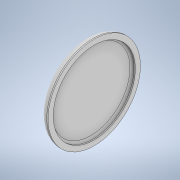
# Autodesk Inventor part: Регулировка-тихая
Saved by Autodesk Inventor 2021 (Build 250183000, 183)
## iProperties
Created: 2023-04-26
Part Number: Регулировка-тихая
Material: Типовые
Document SubType Name: Modeling
Designer: gdevc
Density: 1 g/cm^3
Appearance: По умолчанию
Mass: 33.1576 g
Surface Area: 146.506 cm^2
Volume: 33.1576 cm^3
Author: gdevc
Autodesk Inventor part; units mm, degrees
ref_plane "YZ Plane" through (0, 0, 0) normal (1, 0, 0) x (0, 1, 0)
ref_plane "XZ Plane" through (0, 0, 0) normal (0, 1, 0) x (-1, 0, 0)
ref_plane "XY Plane" through (0, 0, 0) normal (0, 0, 1) x (1, 0, 0)
sketch "Эскиз1" plane through (0, 0, 0) normal (0, 0, 1) x (1, 0, 0)
  line L0 (0, 0) -> (29.6206, 0)
  line L1 (0, 0) -> (0, 38)
  line L2 (2, 40) -> (3.25, 40)
  arc A0 (2, 40) -> (0, 38) centre (2, 38) ccw
  line L3 (3.25, 45) -> (2, 45)
  arc A1 (2, 45) -> (-5, 38) centre (2, 38) ccw
  line L4 (-5, 38) -> (-5, 0)
  line L5 (-5, 0) -> (0, 0)
  line L6 (3.25, 45) -> (3.25, 40)
  dimension "d0" = 80
  dimension "d1" = 2
  dimension "d2" = 90
  dimension "d5" = 8.25
  constraints: 14 end point, 4 point on circle, 3 horizontal, 2 centre point, 2 tangent, 2 vertical, 1 point on line, 1 other
  measures "d0" diameter of L2 L0
  measures "d1" radius of A0
  measures "d2" diameter of L3 L0
  measures "d5" distance between parallel lines of L6 L4
revolve "Вращение1" add sketch "Эскиз1" angle 360 about axis through (0, 0, 0) along (1, 0, 0)
